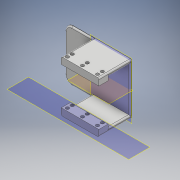
# Autodesk Inventor part: apriltag_head
Saved by Autodesk Inventor 2018 (Build 220112000, 112)
## iProperties
Created: 2020-02-17
Part Number: apriltag_head
Material: Generic
Document SubType Name: Modeling
Designer: bitbots
Density: 1 g/cm^3
Appearance: Default
Author: bitbots
Autodesk Inventor part; units mm, degrees
ref_plane "YZ Plane" through (0, 0, 0) normal (1, 0, 0) x (0, 1, 0)
ref_plane "XZ Plane" through (0, 0, 0) normal (0, 1, 0) x (-1, 0, 0)
ref_plane "Work Plane1" through (0, 0, -55) normal (0, 0, -1) x (1, 0, 0)
sketch "Sketch2" plane through (0, 0, -55) normal (0, 0, -1) x (1, 0, 0)
  circle A0 centre (23, 9) radius 2.35 projected
  circle A1 centre (1, 9) radius 2.35 projected
  circle A2 centre (-21, 9) radius 2.35 projected
  circle A3 centre (-21, 16) radius 2.35 projected
  circle A4 centre (1, 16) radius 2.35 projected
  circle A5 centre (23, 16) radius 2.35 projected
  circle A6 centre (-66, 12.5) radius 1.6 projected
  circle A7 centre (63, 29.65) radius 1.6 projected
  arc A8 (58.9857, 35) -> (49.7248, 32.4349) centre (58.9857, 17) ccw projected
  line L0 (33.2752, 22.5651) -> (49.7248, 32.4349) projected
  arc A9 (24.0143, 20) -> (33.2752, 22.5651) centre (24.0143, 38) ccw projected
  line L1 (-71, 20) -> (24.0143, 20) projected
  arc A10 (-71, 20) -> (-81, 10) centre (-71, 10) ccw projected
  line L2 (-81, 6.5495) -> (-81, 10) projected
  line L3 (-80.0877, 6.5495) -> (-81, 6.5495) projected
  line L4 (81, 6.5495) -> (-80.0877, 6.5495) projected
  line L5 (81, 20) -> (81, 6.5495) projected
  arc A11 (81, 20) -> (66, 35) centre (66, 20) ccw projected
  line L6 (58.9857, 35) -> (66, 35) projected
  line L7 (-21, 16) -> (-26, 16)
  line L8 (-21, 16) -> (-16, 16) construction
  line L9 (-26, 16) -> (-26, 20)
  line L10 (-26, 20) -> (29, 20)
  line L11 (29, 20) -> (29, 6.5495)
  line L12 (29, 6.5495) -> (-26, 6.5495)
  line L13 (-26, 6.5495) -> (-26, 20)
  point P0 (0, 0)
  dimension "d0" = 5
  dimension "d1" = 180
  dimension "d2" = 55
  constraints: 14 end point, 3 horizontal, 2 parallel, 2 perpendicular, 2 point on line, 1 collinear
  measures "d0" distance of L7.start L7.end
  measures "d1" angle of L7 L8
  measures "d2" distance of L11.end L12.end
extrude "Extrusion1" add sketch "Sketch2" along normal blind 10 contours L10 L11 L4 L13 L9 L1
sketch "Sketch3" plane through (-26, -6.5495, -55) normal (0, 1, 0) x (1, 0, 0)
  line L0 (0, 0) -> (0, 10) projected
  line L1 (0, 10) -> (55, 10)
  line L2 (55, 10) -> (55, 5)
  line L3 (55, 5) -> (0, 5)
  line L4 (0, 5) -> (0, 10)
  point P0 (26, -55)
  dimension "d5" = 55
  dimension "d6" = 5
  constraints: 8 end point, 2 parallel, 1 horizontal, 1 perpendicular
  measures "d5" distance of L2.end L3.end
  measures "d6" distance of L1.end L2.end
extrude "Extrusion2" add sketch "Sketch3" along normal blind 35
sketch "Sketch4" plane through (-26, -6.5495, -60) normal (0, 0, 1) x (1, 0, 0)
  line L0 (0, -13.4505) -> (0, 35) projected
  line L1 (0, 35) -> (55, 35)
  line L2 (55, 35) -> (55, 32)
  line L3 (55, 32) -> (0, 32)
  line L4 (0, 32) -> (0, 35)
  point P0 (26, 6.5495)
  dimension "d9" = 55
  dimension "d10" = 3
  constraints: 8 end point, 2 parallel, 1 horizontal, 1 perpendicular
  measures "d9" distance of L2.end L3.end
  measures "d10" distance of L1.end L2.end
ref_plane "Work Plane2" through (-91.43, -48.7723, -27.5) normal (0, 0, 1) x (1, 0, 0)
extrude "Extrusion3" add sketch "Sketch4" along normal up to surface (32.5 mm away)
ref_plane "Work Plane3" through (-26, -6.5495, -27.5) normal (0, 0, 1) x (1, 0, 0)
mirror "Mirror1" about plane through (-26, -6.5495, -27.5) normal (0, 0, 1) of "Extrusion3", "Extrusion2", "Extrusion1"
ref_plane "Work Plane4" through (-26, 25.4505, -55) normal (0, 1, 0) x (1, 0, 0)
sketch "Sketch5" plane through (-26, 25.4505, -55) normal (0, 1, 0) x (1, 0, 0)
  line L0 (55, 5) -> (55, -60) projected
  line L1 (55, -27.5) -> (55, -65)
  line L2 (55, -27.5) -> (92.5, -27.5) construction
  line L3 (55, -65) -> (-40, -65)
  line L4 (-40, -65) -> (-40, 10)
  line L5 (-40, 10) -> (55, 10)
  line L6 (55, 10) -> (55, -65)
  line L7 (55, -65) -> (0, -65) projected
  line L8 (55, 10) -> (0, 10) projected
  line L9 (0, 10) -> (0, -65) projected
  line L10 (-12, 10) -> (-12, -65) construction
  line L11 (-48.9083, -27.5) -> (104.1186, -27.5) construction
  circle A0 centre (-12, -27.5) radius 3
  point P0 (26, -55)
  dimension "d16" = 90
  dimension "d21" = 0
  dimension "d22" = 0
  dimension "d23" = 40
  dimension "d24" = 28
  dimension "d25" = 6
  constraints: 16 end point, 4 point on line, 3 perpendicular, 2 horizontal, 2 midpoint, 2 parallel, 1 centre point, 1 collinear
  measures "d16" angle of L1 L2
  measures "d21" distance between parallel lines of L7 L3
  measures "d22" distance between parallel lines of L8 L5
  measures "d23" distance between parallel lines of L9 L4
  measures "d24" distance between parallel lines of L4 L10
  measures "d25" diameter of A0
extrude "Extrusion4" add sketch "Sketch5" along normal blind 3 contours L0 L1 L3 L9 L5 L6 | L9 L3 L4 L5 | A0
sketch "Sketch6" plane through (-26, 28.4505, -55) normal (0, 1, 0) x (1, 0, 0)
  point P0 (26, -55)
sketch "Sketch7" plane through (-26, 25.4505, -55) normal (0, 1, 0) x (1, 0, 0)
  point P0 (26, -55)
sketch "Sketch8" plane through (-26, 28.4505, -55) normal (0, 1, 0) x (1, 0, 0)
  line L0 (55, 10) -> (-40, 10) projected
  line L1 (-40, -65) -> (55, -65) projected
  line L2 (-12, 10) -> (-12, -65) construction
  line L3 (-40, 10) -> (-40, -65) construction
  line L4 (-40, -27.5) -> (55, -27.5) construction
  line L5 (55, 5) -> (55, -60) construction
  circle A0 centre (-12, -27.5) radius 3
  point P0 (26, -55)
  dimension "d26" = 6
  constraints: 4 end point, 3 midpoint, 3 point on line, 1 centre point, 1 perpendicular
  measures "d26" diameter of A0
extrude "Extrusion5" cut sketch "Sketch8" against normal blind 3 from surface at 0
fillet "Fillet1" radius 0.5 1 edges at (-41, 28.4505, -27.5)
fillet "Fillet2" radius 0.5 1 edges at (-41, 25.4505, -27.5)
fillet "Fillet3" radius 10 2 edges at (-66, 26.9505, 10) (-66, 26.9505, -65)
fillet "Fillet4" radius 2 12 edges at (-26, 9.4505, 5) (-26, 2.7253, 10) (29, 9.4505, 5) (29, 9.4505, -60) (-26, 2.7253, -65) (-26, 9.4505, -60) (-63.0711, 25.4505, -62.0711) (-66, 25.4505, -27.5) (-63.0711, 25.4505, 7.0711) (-41, 25.4505, 10) (-41, 25.4505, -65) (29, 25.4505, -27.5)
fillet "Fillet5" radius 2 2 edges at (29, 4.2253, -65) (29, 4.2253, 10)
fillet "Fillet6" radius 0.5 8 edges at (-63.0711, 28.4505, -62.0711) (-66, 28.4505, -27.5) (-63.0711, 28.4505, 7.0711) (-14.5, 28.4505, 10) (28.4142, 28.4505, 9.4142) (29, 28.4505, -27.5) (28.4142, 28.4505, -64.4142) (-14.5, 28.4505, -65)
body "Solid1"
